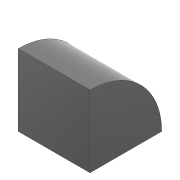
# Autodesk Inventor part: Eihalter_Halter
Saved by Autodesk Inventor 2020 (Build 240168000, 168)
## iProperties
Created: 2022-02-02
Part Number: Eihalter_Halter
Material: Acetalharz, Schwarz
Document SubType Name: Modeling
Designer: Julian Uhl
Density: 1.425 g/cm^3
Appearance: Glatt - Schwarz
Author: Julian Uhl
Autodesk Inventor part; units mm, degrees
ref_plane "YZ Plane" through (0, 0, 0) normal (1, 0, 0) x (0, 1, 0)
ref_plane "XZ Plane" through (0, 0, 0) normal (0, 1, 0) x (-1, 0, 0)
ref_plane "XY Plane" through (0, 0, 0) normal (0, 0, 1) x (1, 0, 0)
sketch "Skizze1" plane through (0, 0, 0) normal (0, 0, 1) x (1, 0, 0)
  line L0 (-9.6, 0) -> (1.6, 0) projected
  line L1 (0, -9.6) -> (0, 1.6) projected
  line L2 (0, 0) -> (-8, 0)
  line L3 (-8, 0) -> (-8, -8)
  line L4 (-8, -8) -> (0, -8)
  line L5 (0, -8) -> (0, 0)
  point P0 (0, -8)
  point P1 (-8, 0)
  point P2 (0, -8)
  dimension "d0" = 8
  dimension "d1" = 8
  constraints: 8 end point, 2 parallel, 1 horizontal, 1 perpendicular
  measures "d0" distance between parallel lines of L0 L4
  measures "d1" distance between parallel lines of L1 L3
extrude "Extrusion1" add sketch "Skizze1" along normal blind 8
fillet "Rundung2" radius 8 1 edges at (-4, 0, 0)
